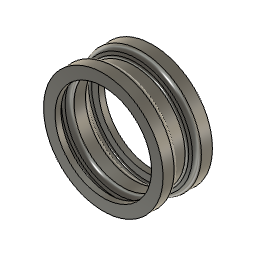
MS Pipe (Autodesk Fusion 360 design; units mm, degrees)
Autodesk Fusion 360 part; units mm, degrees
sketch "Sketch1" plane through (0, 0, 0) normal (0, 0, 1) x (1, 0, 0)
  line L0 (48.0104, 91.141) -> (64.5854, 91.141)
  line L1 (48.0104, 77.441) -> (64.5854, 77.441)
  line L2 (48.0104, 89.491) -> (63.3229, 89.491)
  line L3 (61.3854, 84.291) -> (61.3854, 85.8802)
  line L4 (63.7229, 89.091) -> (63.7229, 88.0796)
  arc A0 (63.7229, 89.091) -> (63.3229, 89.491) centre (63.3229, 89.091) ccw
  line L5 (63.2782, 87.5) -> (62.4601, 87.2808)
  arc A1 (63.2782, 87.5) -> (63.7229, 88.0796) centre (63.1229, 88.0796) ccw
  arc A2 (62.4601, 87.2808) -> (61.3854, 85.8802) centre (62.8354, 85.8802) ccw
  arc A3 (63.5014, 86.6669) -> (64.5854, 88.0796) centre (63.1229, 88.0796) ccw
  line L6 (63.5014, 86.6669) -> (62.6834, 86.4477)
  arc A4 (62.6834, 86.4477) -> (62.2479, 85.8802) centre (62.8354, 85.8802) ccw
  line L7 (62.2479, 84.291) -> (62.2479, 85.8802)
  line L8 (64.5854, 91.141) -> (64.5854, 88.0796)
  line L9 (63.2782, 81.082) -> (62.4601, 81.3012)
  arc A5 (64.5854, 80.5024) -> (63.5014, 81.9151) centre (63.1229, 80.5024) ccw
  line L10 (63.5014, 81.9151) -> (62.6834, 82.1343)
  line L11 (64.5854, 77.441) -> (64.5854, 80.5024)
  arc A6 (63.7229, 80.5024) -> (63.2782, 81.082) centre (63.1229, 80.5024) ccw
  line L12 (48.0104, 79.091) -> (63.3229, 79.091)
  line L13 (63.7229, 79.491) -> (63.7229, 80.5024)
  arc A7 (63.3229, 79.091) -> (63.7229, 79.491) centre (63.3229, 79.491) ccw
  line L14 (48.0104, 77.441) -> (64.5854, 77.441)
  arc A8 (61.3854, 82.7018) -> (62.4601, 81.3012) centre (62.8354, 82.7018) ccw
  line L15 (61.3854, 84.291) -> (61.3854, 82.7018)
  line L16 (62.2479, 84.291) -> (62.2479, 82.7018)
  arc A9 (62.2479, 82.7018) -> (62.6834, 82.1343) centre (62.8354, 82.7018) ccw
  line L17 (48.0104, 91.141) -> (48.0104, 89.491)
  line L18 (48.0104, 79.091) -> (48.0104, 77.441)
  line L19 (61.3854, 79.091) -> (61.3854, 77.441)
  line L20 (61.3854, 89.491) -> (61.3854, 91.141)
  point P0 (63.7229, 89.491)
  point P1 (63.7229, 79.091)
  dimension "d1" = 16.575
  dimension "d2" = 13.7
  dimension "d7" = 15.7125
  dimension "d13" = 0.4
  dimension "d19" = 0.6
  dimension "d20" = 1.45
  constraint coincident P0 L2
  constraint coincident P0 L4
  constraint tangent L2 A0
  constraint tangent L4 A0
  constraint tangent L4 A1
  constraint tangent L5 A1
  constraint tangent L5 A2
  constraint tangent L3 A2
  constraint perpendicular L0 L8
  constraint concentric A1 A3
  constraint parallel L5 L6
  constraint concentric A2 A4
  constraint parallel L3 L7
  constraint tangent A4 L7
  constraint tangent L6 A4
  constraint tangent A3 L6
  constraint perpendicular L0 L17
  constraint perpendicular L14 L18
  constraint coincident L12 L19.start
  constraint coincident L1 L19.end
  constraint perpendicular L1 L19
  constraint coincident L2 L20.start
  constraint coincident L0 L20.end
  constraint perpendicular L0 L20
  measures "d1" distance of L0.start L0.end
  measures "d2" distance of L0.start L1.start
  measures "d7" distance of L2.start P0
  measures "d13" radius of A0
  measures "d19" radius of A1
  measures "d20" radius of A2
revolve "Revolve1" add sketch "Sketch1" angle 360 about axis through (48.0104, 91.141, 0) along (0, -1, 0) contours L0 L1 L2 L3 L4 A0 L5 A1 A2 A3 L6 A4 L7 L8 L9 A5 L10 L11 A6 L12 L13 A7 L14 A8 L15 L16 A9 L19 L20
